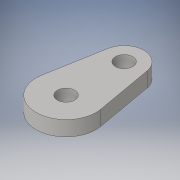
# Autodesk Inventor part: GripperServoHorn
Saved by Autodesk Inventor 2016 (Build 200138000, 138)
## iProperties
Created: 2016-07-08
Part Number: GripperServoHorn
Material: Generic
Document SubType Name: Modeling
Designer: lachesis
Density: 1 g/cm^3
Appearance: Default
Author: lachesis
Autodesk Inventor part; units mm, degrees
ref_plane "YZ Plane" through (0, 0, 0) normal (1, 0, 0) x (0, 1, 0)
ref_plane "XZ Plane" through (0, 0, 0) normal (0, 1, 0) x (-1, 0, 0)
ref_plane "XY Plane" through (0, 0, 0) normal (0, 0, 1) x (1, 0, 0)
sketch "Sketch1" plane through (0, 0, 0) normal (0, 1, 0) x (-1, 0, 0)
  arc A0 (6.2517, -1.1129) -> (-6.2517, -1.1129) centre (0, 0) ccw
  arc A1 (-4.1261, -13.0535) -> (4.1261, -13.0535) centre (0, -12.319) ccw
  line L0 (6.2517, -1.1129) -> (4.1261, -13.0535)
  line L1 (-6.2517, -1.1129) -> (-4.1261, -13.0535)
  dimension "d0" = 22.86
  dimension "d1" = 12.7
  dimension "d2" = 8.382
  constraints: 4 end point, 4 point on circle, 4 tangent, 2 centre point, 1 coincident, 1 vertical alignment
  measures "d1" diameter of A0
  measures "d2" diameter of A1
extrude "Extrusion1" add sketch "Sketch1" along normal blind 3.175
sketch "Sketch2" plane through (0, 3.175, 0) normal (0, 1, 0) x (1, 0, 0)
  arc A0 (-6.2517, 1.1129) -> (6.2517, 1.1129) centre (0, 0) ccw projected
  arc A1 (4.1261, 13.0535) -> (-4.1261, 13.0535) centre (0, 12.319) ccw projected
  constraints: 2 coincident
hole "Hole1" at (0, 3.175, 0) at (0, 3.175, -12.319) direction (0, -1, 0) diameter 3.683 end through all
body "Solid1"
